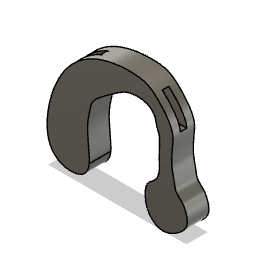
HearingAidWithSlits v3 (Autodesk Fusion 360 design; units mm, degrees)
Autodesk Fusion 360 part; units mm, degrees
sketch "Sketch1" plane through (0, 0, 0) normal (0, 0, 1) x (1, 0, 0)
  spline S0 degree 5 poles (28.5, 11) (28.5862, 11.1307) (28.7498, 11.3926) (28.9684, 11.787) (29.2063, 12.316) (29.416, 12.984) (29.5428, 13.6633) (29.5965, 14.3631) (29.593, 15.0979) (29.5495, 15.884) (29.4827, 16.7367) (29.4039, 17.6667) (29.318, 18.6782) (29.2264, 19.7703) (29.1286, 20.9368) (29.0259, 22.1679) (28.9227, 23.4502) (28.8298, 24.7675) (28.7627, 26.1019) (28.7374, 27.4344) (28.7678, 28.7458) (28.8621, 30.0172) (29.0194, 31.2315) (29.2267, 32.3734) (29.4563, 33.431) (29.6779, 34.3975) (29.867, 35.2734) (30.0152, 36.0681) (30.1401, 36.8025) (30.2936, 37.51) (30.5433, 38.2288) (30.9551, 38.9936) (31.5756, 39.8277) (32.414, 40.7357) (33.4508, 41.707) (34.6453, 42.7205) (35.9429, 43.7482) (37.2834, 44.7593) (38.6083, 45.7247) (39.8685, 46.6203) (41.033, 47.4322) (42.0896, 48.156) (43.0414, 48.7943) (43.9052, 49.3542) (44.7089, 49.8453) (45.4886, 50.2776) (46.2877, 50.6586) (47.1506, 50.9923) (48.1154, 51.2783) (49.2064, 51.5106) (50.4273, 51.677) (51.7522, 51.7572) (53.1277, 51.7263) (54.4866, 51.5626) (55.7574, 51.254) (56.8759, 50.8054) (57.7955, 50.2448) (58.4992, 49.6324) (59.0064, 49.0596) (59.3585, 48.5993) (59.6077, 48.2726) (59.8039, 47.9887) (59.9869, 47.5705) (60.1852, 46.8908) (60.413, 45.9742) (60.673, 44.9382) (60.9576, 43.9317) (61.2518, 43.0801) (61.5345, 42.416) (61.7816, 41.8542) (61.972, 41.2627) (62.0922, 40.5095) (62.1433, 39.529) (62.1386, 38.3242) (62.099, 36.9427) (62.0479, 35.4617) (62.0068, 33.9677) (61.9911, 32.541) (62.0045, 31.2343) (62.0369, 30.0632) (62.0695, 29.0179) (62.0781, 28.071) (62.0373, 27.1871) (61.9244, 26.3311) (61.7237, 25.4784) (61.426, 24.6148) (61.1065, 23.9092) (60.8205, 23.3707) (60.6093, 23.0075) (60.4985, 22.8249) knots 0 0 0 0 0 0 0.01176471 0.02352941 0.03529412 0.04705882 0.05882353 0.07058824 0.08235294 0.09411765 0.10588235 0.11764706 0.12941176 0.14117647 0.15294118 0.16470588 0.17647059 0.18823529 0.2 0.21176471 0.22352941 0.23529412 0.24705882 0.25882353 0.27058824 0.28235294 0.29411765 0.30588235 0.31764706 0.32941176 0.34117647 0.35294118 0.36470588 0.37647059 0.38823529 0.4 0.41176471 0.42352941 0.43529412 0.44705882 0.45882353 0.47058824 0.48235294 0.49411765 0.50588235 0.51764706 0.52941176 0.54117647 0.55294118 0.56470588 0.57647059 0.58823529 0.6 0.61176471 0.62352941 0.63529412 0.64705882 0.65882353 0.67058824 0.68235294 0.69411765 0.70588235 0.71764706 0.72941176 0.74117647 0.75294118 0.76470588 0.77647059 0.78823529 0.8 0.81176471 0.82352941 0.83529412 0.84705882 0.85882353 0.87058824 0.88235294 0.89411765 0.90588235 0.91764706 0.92941176 0.94117647 0.95294118 0.96470588 0.97647059 0.98823529 1 1 1 1 1 1
  spline S1 degree 5 poles (60.4985, 22.8249) (60.3549, 22.6726) (60.0693, 22.377) (59.6455, 21.9608) (59.0896, 21.4604) (58.4119, 20.9118) (57.756, 20.4022) (57.1316, 19.849) (56.5549, 19.1446) (56.0501, 18.1928) (55.6523, 16.9462) (55.4057, 15.424) (55.3562, 13.6895) (55.5448, 11.8383) (56.0004, 9.9805) (56.7338, 8.2273) (57.7286, 6.6733) (58.9462, 5.392) (60.334, 4.4354) (61.8334, 3.8329) (63.3874, 3.59) (64.9488, 3.6872) (66.4881, 4.0785) (67.9861, 4.7031) (69.4278, 5.496) (70.795, 6.4) (72.06, 7.3753) (73.1767, 8.4142) (74.0827, 9.5397) (74.7178, 10.7813) (75.0394, 12.1554) (75.0367, 13.6471) (74.7519, 15.1831) (74.2753, 16.6386) (73.7119, 17.8865) (73.151, 18.8399) (72.6413, 19.4878) (72.1481, 19.958) (71.5992, 20.4402) (70.9625, 21.0598) (70.3256, 21.7469) (69.8191, 22.3627) (69.5251, 22.8464) (69.3776, 23.3816) (69.2357, 24.2413) (69.0073, 25.5313) (68.6986, 27.1048) (68.3636, 28.707) (68.0754, 30.0761) (67.8926, 31.0446) (67.8172, 31.6817) (67.7997, 32.2569) (67.7902, 33.0466) (67.7823, 34.1612) (67.8004, 35.5694) (67.8742, 37.1654) (68.0192, 38.8188) (68.2111, 40.4364) (68.3719, 42.0047) (68.3975, 43.5571) (68.1795, 45.1512) (67.6307, 46.8414) (66.7063, 48.6561) (65.4328, 50.5667) (63.9137, 52.4808) (62.2938, 54.2759) (60.7335, 55.8247) (59.3792, 57.023) (58.3337, 57.8187) (57.6311, 58.2337) (57.1982, 58.4065) (56.8675, 58.553) (56.4594, 58.7925) (55.8244, 59.1018) (54.8607, 59.4258) (53.5261, 59.7227) (51.8219, 59.9561) (49.7838, 60.0964) (47.4695, 60.1179) (44.9486, 59.9985) (42.2902, 59.7176) (39.5543, 59.2556) (36.7936, 58.5948) (34.053, 57.7195) (31.3713, 56.6175) (28.7805, 55.2799) (26.3074, 53.7025) (23.9733, 51.8861) (21.7952, 49.8375) (19.7856, 47.5697) (17.9535, 45.1033) (16.3051, 42.4659) (14.8437, 39.6912) (13.5712, 36.8169) (12.4883, 33.8842) (11.5953, 30.9357) (10.8926, 28.0145) (10.3814, 25.1631) (10.0647, 22.4213) (9.9472, 19.8257) (10.0369, 17.4077) (10.3448, 15.1925) (10.882, 13.2) (11.6564, 11.445) (12.6695, 9.9381) (13.9129, 8.6859) (15.3655, 7.6923) (16.9895, 6.9586) (18.7294, 6.484) (20.519, 6.2665) (22.2872, 6.3032) (23.964, 6.5906) (25.4862, 7.1255) (26.8045, 7.9049) (27.8865, 8.927) (28.713, 10.1906) (29.162, 11.3941) (29.3779, 12.405) (29.4683, 13.127) (29.5, 13.5) knots 0 0 0 0 0 0 0.00869565 0.0173913 0.02608696 0.03478261 0.04347826 0.05217391 0.06086957 0.06956522 0.07826087 0.08695652 0.09565217 0.10434783 0.11304348 0.12173913 0.13043478 0.13913043 0.14782609 0.15652174 0.16521739 0.17391304 0.1826087 0.19130435 0.2 0.20869565 0.2173913 0.22608696 0.23478261 0.24347826 0.25217391 0.26086957 0.26956522 0.27826087 0.28695652 0.29565217 0.30434783 0.31304348 0.32173913 0.33043478 0.33913043 0.34782609 0.35652174 0.36521739 0.37391304 0.3826087 0.39130435 0.4 0.40869565 0.4173913 0.42608696 0.43478261 0.44347826 0.45217391 0.46086957 0.46956522 0.47826087 0.48695652 0.49565217 0.50434783 0.51304348 0.52173913 0.53043478 0.53913043 0.54782609 0.55652174 0.56521739 0.57391304 0.5826087 0.59130435 0.6 0.60869565 0.6173913 0.62608696 0.63478261 0.64347826 0.65217391 0.66086957 0.66956522 0.67826087 0.68695652 0.69565217 0.70434783 0.71304348 0.72173913 0.73043478 0.73913043 0.74782609 0.75652174 0.76521739 0.77391304 0.7826087 0.79130435 0.8 0.80869565 0.8173913 0.82608696 0.83478261 0.84347826 0.85217391 0.86086957 0.86956522 0.87826087 0.88695652 0.89565217 0.90434783 0.91304348 0.92173913 0.93043478 0.93913043 0.94782609 0.95652174 0.96521739 0.97391304 0.9826087 0.99130435 1 1 1 1 1 1
  point P0 (29.5, 13.5)
  point P1 (29.5, 16.5)
  point P2 (29, 22.5)
  point P3 (29, 31)
  point P4 (30, 36)
  point P5 (31, 39)
  point P6 (39, 46)
  point P7 (45, 50)
  point P8 (49.7706, 51.576)
  point P9 (57.5539, 50.3613)
  point P10 (59.4885, 48.4267)
  point P11 (59.9834, 47.5269)
  point P12 (61.1532, 43.3878)
  point P13 (62, 41)
  point P14 (62, 33)
  point P15 (62, 27)
  point P16 (58.1753, 20.7274)
  point P17 (56.2497, 18.5073)
  point P18 (56.2497, 9.5)
  point P19 (63.3958, 3.6745)
  point P20 (71.5149, 6.9766)
  point P21 (75, 13)
  point P22 (73, 19)
  point P23 (71.5149, 20.5325)
  point P24 (69.8148, 22.4116)
  point P25 (69.2833, 23.9601)
  point P26 (68, 30.5)
  point P27 (67.7998, 32.4162)
  point P28 (68, 38.5)
  point P29 (67, 48)
  point P30 (58, 58)
  point P31 (57, 58.5)
  point P32 (56, 59)
  point P33 (45.5, 60)
  point P34 (20.5917, 48.4267)
  point P35 (10, 20)
  point P36 (15, 8)
  point P37 (25, 7)
  constraint coincident P0 S1.end
extrude "Extrude1" add sketch "Sketch1" along normal blind 10
sketch "Sketch2" plane through (0, 0, 0) normal (1, 0, 0) x (0, 0, -1)
sketch "Sketch3" plane through (0, 0, 0) normal (1, 0, 0) x (0, 0, -1)
  line L0 (-6.5, 56.5417) -> (-3.5, 56.5417)
  line L1 (-3.5, 56.5417) -> (-3.5, 43.9417)
  line L2 (-3.5, 43.9417) -> (-6.5, 43.9417)
  line L3 (-6.5, 43.9417) -> (-6.5, 56.5417)
  line L4 (-10, 3.6663) -> (-10, 60.092)
  dimension "d3" = 3
  dimension "d4" = 12.6
  dimension "d5" = 3.5
  constraint horizontal L0
  constraint vertical L1
  constraint horizontal L2
  constraint vertical L3
  measures "d3" distance of L0.start L0.end
  measures "d4" distance of L0.end L1.end
  measures "d5" distance of L3 L4
extrude "Extrude2" cut sketch "Sketch3" along normal blind 135
